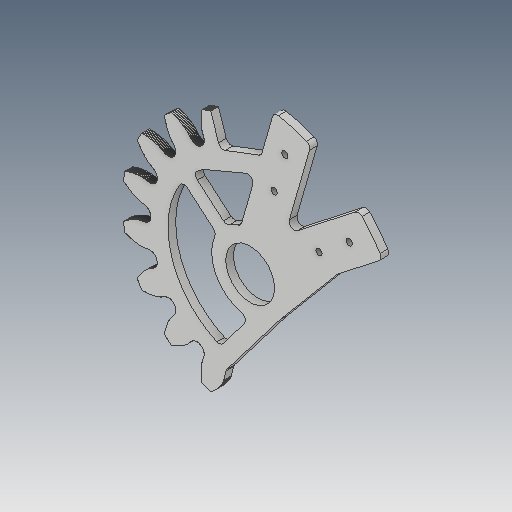
# Autodesk Inventor part: m5-18
Saved by Autodesk Inventor 2019.4 (Build 234330000, 330)
## iProperties
Created: 2019-06-11
Part Number: m5-18
Material: Generic
Document SubType Name: Modeling
Designer: AzLIer
Density: 1 g/cm^3
Appearance: Default
Mass: 10.3101 g
Surface Area: 90.7911 cm^2
Volume: 10.3101 cm^3
Autodesk Inventor part; units mm, degrees
(part 1 of 5)
ref_plane "YZ Plane" through (0, 0, 0) normal (1, 0, 0) x (0, 1, 0)
ref_plane "XZ Plane" through (0, 0, 0) normal (0, 1, 0) x (-1, 0, 0)
ref_plane "XY Plane" through (0, 0, 0) normal (0, 0, 1) x (1, 0, 0)
sketch "スケッチ1" plane through (0, 0, 0) normal (0, 0, 1) x (1, 0, 0)
  circle A0 centre (0, 0) radius 45 construction
  line L0 (-54, 0) -> (54, 0) construction
  line L1 (0, -54) -> (0, 54) construction
  line L2 (38.75, 0) -> (38.75, 0.0554)
  line L3 (38.75, 0.0554) -> (38.7498, 0.1108)
  line L4 (38.7498, 0.1108) -> (38.7496, 0.1663)
  line L5 (38.7496, 0.1663) -> (38.7494, 0.2217)
  line L6 (38.7494, 0.2217) -> (38.749, 0.2771)
  line L7 (38.749, 0.2771) -> (38.7743, 0.6234)
  line L8 (38.7743, 0.6234) -> (38.8288, 0.891)
  line L9 (38.8288, 0.891) -> (38.9042, 1.1194)
  line L10 (38.9042, 1.1194) -> (38.997, 1.3323)
  line L11 (38.997, 1.3323) -> (39.1059, 1.5242)
  line L12 (39.1059, 1.5242) -> (39.2291, 1.7067)
  line L13 (39.2291, 1.7067) -> (39.366, 1.8725)
  line L14 (39.366, 1.8725) -> (39.5158, 2.0289)
  line L15 (39.5158, 2.0289) -> (39.6781, 2.1727)
  line L16 (39.6781, 2.1727) -> (39.8523, 2.3033)
  line L17 (39.8523, 2.3033) -> (40.0379, 2.4272)
  line L18 (40.0379, 2.4272) -> (40.2348, 2.5371)
  line L19 (40.2348, 2.5371) -> (40.4428, 2.6351)
  line L20 (40.4428, 2.6351) -> (40.661, 2.7274)
  line L21 (40.661, 2.7274) -> (40.8898, 2.8078)
  line L22 (40.8898, 2.8078) -> (41.1289, 2.8764)
  line L23 (41.1289, 2.8764) -> (41.3781, 2.9334)
  line L24 (41.3781, 2.9334) -> (41.6367, 2.9845)
  line L25 (41.6367, 2.9845) -> (41.9049, 3.0266)
  line L26 (41.9049, 3.0266) -> (42.1825, 3.0578)
  line L27 (42.1825, 3.0578) -> (42.555, 3.1194)
  line L28 (42.555, 3.1194) -> (42.9254, 3.2087)
  line L29 (42.9254, 3.2087) -> (43.2942, 3.3167)
  line L30 (43.2942, 3.3167) -> (43.6617, 3.4402)
  line L31 (43.6617, 3.4402) -> (44.0279, 3.5774)
  line L32 (44.0279, 3.5774) -> (44.3927, 3.7271)
  line L33 (44.3927, 3.7271) -> (44.7563, 3.8884)
  line L34 (44.7563, 3.8884) -> (45.1184, 4.0607)
  line L35 (45.1184, 4.0607) -> (45.4792, 4.2434)
  line L36 (45.4792, 4.2434) -> (45.8385, 4.4362)
  line L37 (45.8385, 4.4362) -> (46.1963, 4.6386)
  line L38 (46.1963, 4.6386) -> (46.5526, 4.8504)
  line L39 (46.5526, 4.8504) -> (46.9072, 5.0713)
  line L40 (46.9072, 5.0713) -> (47.2601, 5.3011)
  line L41 (47.2601, 5.3011) -> (47.6113, 5.5395)
  line L42 (47.6113, 5.5395) -> (47.9606, 5.7865)
  line L43 (47.9606, 5.7865) -> (48.308, 6.0419)
  line L44 (48.308, 6.0419) -> (48.6534, 6.3055)
  line L45 (48.6534, 6.3055) -> (48.9968, 6.5771)
  line L46 (48.9968, 6.5771) -> (49.338, 6.8568)
  line L47 (49.338, 6.8568) -> (49.2867, 7.2162)
  line L48 (49.2867, 7.2162) -> (49.2328, 7.5752)
  line L49 (49.2328, 7.5752) -> (49.1763, 7.9338)
  line L50 (49.1763, 7.9338) -> (49.1172, 8.292)
  line L51 (49.1172, 8.292) -> (49.0554, 8.6498)
  circle A1 centre (0, 0) radius 45 construction
  line L52 (38.75, 0) -> (38.75, -0.0554)
  line L53 (38.75, -0.0554) -> (38.7498, -0.1108)
  line L54 (38.7498, -0.1108) -> (38.7496, -0.1663)
  line L55 (38.7496, -0.1663) -> (38.7494, -0.2217)
  line L56 (38.7494, -0.2217) -> (38.749, -0.2771)
  line L57 (38.749, -0.2771) -> (38.7743, -0.6234)
  line L58 (38.7743, -0.6234) -> (38.8288, -0.891)
  line L59 (38.8288, -0.891) -> (38.9042, -1.1194)
  line L60 (38.9042, -1.1194) -> (38.997, -1.3323)
  line L61 (38.997, -1.3323) -> (39.1059, -1.5242)
  line L62 (39.1059, -1.5242) -> (39.2291, -1.7067)
  line L63 (39.2291, -1.7067) -> (39.366, -1.8725)
  line L64 (39.366, -1.8725) -> (39.5158, -2.0289)
  line L65 (39.5158, -2.0289) -> (39.6781, -2.1727)
  line L66 (39.6781, -2.1727) -> (39.8523, -2.3033)
  line L67 (39.8523, -2.3033) -> (40.0379, -2.4272)
  line L68 (40.0379, -2.4272) -> (40.2348, -2.5371)
  line L69 (40.2348, -2.5371) -> (40.4428, -2.6351)
  line L70 (40.4428, -2.6351) -> (40.661, -2.7274)
  line L71 (40.661, -2.7274) -> (40.8898, -2.8078)
  line L72 (40.8898, -2.8078) -> (41.1289, -2.8764)
  line L73 (41.1289, -2.8764) -> (41.3781, -2.9334)
  line L74 (41.3781, -2.9334) -> (41.6367, -2.9845)
  line L75 (41.6367, -2.9845) -> (41.9049, -3.0266)
  line L76 (41.9049, -3.0266) -> (42.1825, -3.0578)
  line L77 (42.1825, -3.0578) -> (42.555, -3.1194)
  line L78 (42.555, -3.1194) -> (42.9254, -3.2087)
  line L79 (42.9254, -3.2087) -> (43.2942, -3.3167)
  line L80 (43.2942, -3.3167) -> (43.6617, -3.4402)
  line L81 (43.6617, -3.4402) -> (44.0279, -3.5774)
  line L82 (44.0279, -3.5774) -> (44.3927, -3.7271)
  line L83 (44.3927, -3.7271) -> (44.7563, -3.8884)
  line L84 (44.7563, -3.8884) -> (45.1184, -4.0607)
  line L85 (45.1184, -4.0607) -> (45.4792, -4.2434)
  line L86 (45.4792, -4.2434) -> (45.8385, -4.4362)
  line L87 (45.8385, -4.4362) -> (46.1963, -4.6386)
  line L88 (46.1963, -4.6386) -> (46.5526, -4.8504)
  line L89 (46.5526, -4.8504) -> (46.9072, -5.0713)
  line L90 (46.9072, -5.0713) -> (47.2601, -5.3011)
  line L91 (47.2601, -5.3011) -> (47.6113, -5.5395)
  line L92 (47.6113, -5.5395) -> (47.9606, -5.7865)
  line L93 (47.9606, -5.7865) -> (48.308, -6.0419)
  line L94 (48.308, -6.0419) -> (48.6534, -6.3055)
  line L95 (48.6534, -6.3055) -> (48.9968, -6.5771)
  line L96 (48.9968, -6.5771) -> (49.338, -6.8568)
  line L97 (49.338, -6.8568) -> (49.2867, -7.2162)
  line L98 (49.2867, -7.2162) -> (49.2328, -7.5752)
  line L99 (49.2328, -7.5752) -> (49.1763, -7.9338)
  line L100 (49.1763, -7.9338) -> (49.1172, -8.292)
  line L101 (49.1172, -8.292) -> (49.0554, -8.6498)
  line L102 (38.0283, 11.529) -> (38.2367, 11.4659)
  line L103 (38.2367, 11.4659) -> (38.4534, 11.4129)
  line L104 (38.4534, 11.4129) -> (38.6761, 11.377)
  line L105 (38.6761, 11.377) -> (38.905, 11.3561)
  line L106 (39.1417, 11.344) -> (39.3842, 11.3467)
  line L107 (39.3842, 11.3467) -> (39.6323, 11.364)
  line L108 (39.6323, 11.364) -> (39.886, 11.3956)
  line L109 (39.886, 11.3956) -> (40.1465, 11.4361)
  line L110 (40.1465, 11.4361) -> (40.4129, 11.4882)
  line L111 (36.4131, 13.2533) -> (36.3941, 13.3053)
  line L112 (36.3941, 13.3053) -> (36.375, 13.3574)
  line L113 (36.375, 13.3574) -> (36.3559, 13.4094)
  line L114 (36.3559, 13.4094) -> (36.3367, 13.4614)
  line L115 (40.6845, 11.5538) -> (41.0555, 11.6234)
  circle A2 centre (0, 0) radius 45 construction
  circle A3 centre (0, 0) radius 45 construction
  line L116 (36.3367, 13.4614) -> (36.3174, 13.5133)
  line L117 (36.3174, 13.5133) -> (36.2227, 13.8474)
  line L118 (36.2227, 13.8474) -> (36.1824, 14.1175)
  line L119 (36.1824, 14.1175) -> (36.1751, 14.3579)
  line L120 (36.1751, 14.3579) -> (36.1896, 14.5898)
  line L121 (36.1896, 14.5898) -> (36.2262, 14.8073)
  line L122 (36.2262, 14.8073) -> (36.2795, 15.0209)
  line L123 (36.2795, 15.0209) -> (36.3516, 15.2235)
  line L124 (36.3516, 15.2235) -> (36.4388, 15.4218)
  line L125 (36.4388, 15.4218) -> (36.5421, 15.6124)
  line L126 (36.5421, 15.6124) -> (36.6611, 15.7947)
  line L127 (36.6611, 15.7947) -> (36.7931, 15.9746)
  line L128 (36.7931, 15.9746) -> (36.9406, 16.1452)
  line L129 (36.9406, 16.1452) -> (37.1025, 16.3084)
  line L130 (37.1025, 16.3084) -> (37.2761, 16.4698)
  line L131 (40.4129, 11.4882) -> (40.6845, 11.5538)
  line L132 (37.2761, 16.4698) -> (37.4636, 16.6236)
  line L133 (37.4636, 16.6236) -> (37.6648, 16.7698)
  line L134 (37.6648, 16.7698) -> (37.8794, 16.9086)
  line L135 (37.8794, 16.9086) -> (38.105, 17.0451)
  line L136 (38.3425, 17.1764) -> (38.5928, 17.3007)
  line L137 (38.105, 17.0451) -> (38.3425, 17.1764)
  line L138 (38.905, 11.3561) -> (39.1417, 11.344)
  line L139 (38.5928, 17.3007) -> (38.9217, 17.4859)
  line L140 (38.9217, 17.4859) -> (39.2392, 17.6965)
  line L141 (39.5489, 17.9241) -> (39.852, 18.1659)
  line L142 (39.852, 18.1659) -> (40.1491, 18.4201)
  line L143 (40.1491, 18.4201) -> (40.4408, 18.6855)
  line L144 (39.2392, 17.6965) -> (39.5489, 17.9241)
  line L145 (37.8267, 11.6087) -> (38.0283, 11.529)
  line L146 (37.447, 11.8133) -> (37.6324, 11.7044)
  line L147 (37.6324, 11.7044) -> (37.8267, 11.6087)
  line L148 (40.7272, 18.9615) -> (41.0086, 19.2472)
  line L149 (42.5969, 21.1453) -> (42.8453, 21.4895)
  line L150 (42.3439, 20.8086) -> (42.5969, 21.1453)
  line L151 (42.0862, 20.4798) -> (42.3439, 20.8086)
  line L152 (41.8239, 20.1589) -> (42.0862, 20.4798)
  line L153 (41.5569, 19.8464) -> (41.8239, 20.1589)
  line L154 (41.2851, 19.5423) -> (41.5569, 19.8464)
  line L155 (41.0086, 19.2472) -> (41.2851, 19.5423)
  line L156 (42.8453, 21.4895) -> (43.0891, 21.841)
  line L157 (43.0891, 21.841) -> (43.3282, 22.1998)
  line L158 (43.3282, 22.1998) -> (43.5626, 22.5656)
  line L159 (43.5626, 22.5656) -> (43.7924, 22.9383)
  line L160 (43.7924, 22.9383) -> (44.0174, 23.3178)
  line L161 (44.0174, 23.3178) -> (43.8463, 23.638)
  line L162 (43.8463, 23.638) -> (43.6728, 23.957)
  line L163 (43.6728, 23.957) -> (43.4971, 24.2746)
  line L164 (43.4971, 24.2746) -> (43.319, 24.591)
  line L165 (43.319, 24.591) -> (43.1386, 24.9061)
  line L166 (40.4408, 18.6855) -> (40.7272, 18.9615)
  line L167 (37.2688, 11.9427) -> (37.447, 11.8133)
  line L168 (42.9903, 11.6809) -> (43.387, 11.6536)
  line L169 (42.5962, 11.6968) -> (42.9903, 11.6809)
  line L170 (42.2052, 11.7005) -> (42.5962, 11.6968)
  line L171 (41.8176, 11.6908) -> (42.2052, 11.7005)
  line L172 (41.4341, 11.6662) -> (41.8176, 11.6908)
  line L173 (41.0555, 11.6234) -> (41.4341, 11.6662)
  line L174 (43.387, 11.6536) -> (43.7863, 11.6156)
  line L175 (43.7863, 11.6156) -> (44.1878, 11.5673)
  line L176 (46.6346, 11.0786) -> (47.0473, 10.9659)
  line L177 (46.223, 11.1825) -> (46.6346, 11.0786)
  line L178 (45.8128, 11.2778) -> (46.223, 11.1825)
  line L179 (45.4041, 11.3641) -> (45.8128, 11.2778)
  line L180 (44.9969, 11.4412) -> (45.4041, 11.3641)
  line L181 (44.5914, 11.509) -> (44.9969, 11.4412)
  line L182 (44.1878, 11.5673) -> (44.5914, 11.509)
  line L183 (47.0473, 10.9659) -> (47.4611, 10.8448)
  line L184 (47.8758, 10.7152) -> (48.2914, 10.5774)
  line L185 (48.2914, 10.5774) -> (48.7077, 10.4313)
  line L186 (48.7077, 10.4313) -> (48.7824, 10.0761)
  line L187 (48.7824, 10.0761) -> (48.8546, 9.7203)
  line L188 (48.8546, 9.7203) -> (48.9241, 9.3639)
  line L189 (48.9241, 9.3639) -> (48.9911, 9.0071)
  line L190 (48.9911, 9.0071) -> (49.0554, 8.6498)
  line L191 (47.4611, 10.8448) -> (47.8758, 10.7152)
  line L192 (37.1009, 12.0858) -> (37.2688, 11.9427)
  line L193 (36.9408, 12.2541) -> (37.1009, 12.0858)
  line L194 (36.7919, 12.4429) -> (36.9408, 12.2541)
  line L195 (36.6492, 12.6758) -> (36.7919, 12.4429)
  line L196 (36.5069, 12.9926) -> (36.6492, 12.6758)
  line L197 (36.4883, 13.0448) -> (36.5069, 12.9926)
  line L198 (36.4696, 13.0969) -> (36.4883, 13.0448)
  line L199 (36.4508, 13.1491) -> (36.4696, 13.0969)
  line L200 (36.432, 13.2012) -> (36.4508, 13.1491)
  line L201 (36.4131, 13.2533) -> (36.432, 13.2012)
  line L202 (31.7918, 23.8401) -> (32.0092, 23.8521)
  line L203 (32.0092, 23.8521) -> (32.231, 23.8765)
  line L204 (32.231, 23.8765) -> (32.4525, 23.9189)
  line L205 (32.4525, 23.9189) -> (32.6748, 23.9775)
  line L206 (32.9013, 24.0471) -> (33.1282, 24.1326)
  line L207 (33.1282, 24.1326) -> (33.3555, 24.2337)
  line L208 (33.3555, 24.2337) -> (33.583, 24.3502)
  line L209 (33.583, 24.3502) -> (33.814, 24.4773)
  line L210 (33.814, 24.4773) -> (34.0465, 24.6174)
  line L211 (29.6842, 24.908) -> (29.6486, 24.9504)
  line L212 (29.6486, 24.9504) -> (29.6129, 24.9928)
  line L213 (29.6129, 24.9928) -> (29.5771, 25.0351)
  line L214 (29.5771, 25.0351) -> (29.5412, 25.0774)
  line L215 (34.2792, 24.772) -> (34.6041, 24.9642)
  circle A4 centre (0, 0) radius 45 construction
  circle A5 centre (0, 0) radius 45 construction
  line L216 (29.5412, 25.0774) -> (29.5054, 25.1196)
  line L217 (29.5054, 25.1196) -> (29.3021, 25.4012)
  line L218 (29.3021, 25.4012) -> (29.1718, 25.6412)
  line L219 (29.1718, 25.6412) -> (29.0828, 25.8646)
  line L220 (29.0828, 25.8646) -> (29.0171, 26.0875)
  line L221 (29.0171, 26.0875) -> (28.9771, 26.3044)
  line L222 (28.9771, 26.3044) -> (28.9541, 26.5234)
  line L223 (28.9541, 26.5234) -> (28.9525, 26.7384)
  line L224 (28.9525, 26.7384) -> (28.9667, 26.9545)
  line L225 (28.9667, 26.9545) -> (28.9985, 27.169)
  line L226 (28.9985, 27.169) -> (29.0481, 27.381)
  line L227 (29.0481, 27.381) -> (29.1106, 27.5952)
  line L228 (29.1106, 27.5952) -> (29.1908, 27.806)
  line L229 (29.1908, 27.806) -> (29.2872, 28.0147)
  line L230 (29.2872, 28.0147) -> (29.395, 28.2257)
  line L231 (34.0465, 24.6174) -> (34.2792, 24.772)
  line L232 (29.395, 28.2257) -> (29.5186, 28.4343)
  line L233 (29.5186, 28.4343) -> (29.6577, 28.6406)
  line L234 (29.6577, 28.6406) -> (29.8119, 28.8444)
  line L235 (29.8119, 28.8444) -> (29.9772, 29.0498)
  line L236 (30.1555, 29.2545) -> (30.3482, 29.4569)
  line L237 (29.9772, 29.0498) -> (30.1555, 29.2545)
  line L238 (32.6748, 23.9775) -> (32.9013, 24.0471)
  line L239 (30.3482, 29.4569) -> (30.5939, 29.7434)
  line L240 (30.5939, 29.7434) -> (30.8202, 30.0499)
  line L241 (31.0334, 30.3697) -> (31.2355, 30.7005)
  line L242 (31.2355, 30.7005) -> (31.4278, 31.041)
  line L243 (31.4278, 31.041) -> (31.6111, 31.3902)
  line L244 (30.8202, 30.0499) -> (31.0334, 30.3697)
  line L245 (31.575, 23.8461) -> (31.7918, 23.8401)
  line L246 (31.1483, 23.9085) -> (31.3597, 23.8696)
  line L247 (31.3597, 23.8696) -> (31.575, 23.8461)
  line L248 (31.7858, 31.7475) -> (31.9525, 32.1123)
  line L249 (32.7959, 34.4391) -> (32.9116, 34.8475)
  line L250 (32.6732, 34.0362) -> (32.7959, 34.4391)
  line L251 (32.5436, 33.639) -> (32.6732, 34.0362)
  line L252 (32.4068, 33.2478) -> (32.5436, 33.639)
  line L253 (32.2628, 32.8628) -> (32.4068, 33.2478)
  line L254 (32.1115, 32.4841) -> (32.2628, 32.8628)
  line L255 (31.9525, 32.1123) -> (32.1115, 32.4841)
  line L256 (32.9116, 34.8475) -> (33.0204, 35.2612)
  line L257 (33.0204, 35.2612) -> (33.1224, 35.6801)
  line L258 (33.1224, 35.6801) -> (33.2176, 36.1041)
  line L259 (33.2176, 36.1041) -> (33.306, 36.5329)
  line L260 (33.306, 36.5329) -> (33.3877, 36.9664)
  line L261 (33.3877, 36.9664) -> (33.1173, 37.2088)
  line L262 (33.1173, 37.2088) -> (32.8453, 37.4492)
  line L263 (32.8453, 37.4492) -> (32.5715, 37.6876)
  line L264 (32.5715, 37.6876) -> (32.2959, 37.924)
  line L265 (32.2959, 37.924) -> (32.0186, 38.1583)
  line L266 (31.6111, 31.3902) -> (31.7858, 31.7475)
  line L267 (30.9366, 23.9692) -> (31.1483, 23.9085)
  line L268 (36.4025, 25.68) -> (36.7847, 25.7901)
  line L269 (36.0268, 25.5601) -> (36.4025, 25.68)
  line L270 (35.6581, 25.4299) -> (36.0268, 25.5601)
  line L271 (35.2972, 25.2883) -> (35.6581, 25.4299)
  line L272 (34.9452, 25.1339) -> (35.2972, 25.2883)
  line L273 (34.6041, 24.9642) -> (34.9452, 25.1339)
  line L274 (36.7847, 25.7901) -> (37.1729, 25.8909)
  line L275 (37.1729, 25.8909) -> (37.5667, 25.9828)
  line L276 (40.0331, 26.3604) -> (40.4594, 26.3957)
  line L277 (39.6108, 26.3174) -> (40.0331, 26.3604)
  line L278 (39.1928, 26.2665) -> (39.6108, 26.3174)
  line L279 (38.7791, 26.2078) -> (39.1928, 26.2665)
  line L280 (38.3701, 26.1411) -> (38.7791, 26.2078)
  line L281 (37.9659, 26.0661) -> (38.3701, 26.1411)
  line L282 (37.5667, 25.9828) -> (37.9659, 26.0661)
  line L283 (40.4594, 26.3957) -> (40.8897, 26.4234)
  line L284 (41.3237, 26.4435) -> (41.7614, 26.4561)
  line L285 (41.7614, 26.4561) -> (42.2025, 26.4613)
  line L286 (42.2025, 26.4613) -> (42.3943, 26.153)
  line L287 (42.3943, 26.153) -> (42.5838, 25.8433)
  line L288 (42.5838, 25.8433) -> (42.771, 25.5322)
  line L289 (42.771, 25.5322) -> (42.9559, 25.2198)
  line L290 (42.9559, 25.2198) -> (43.1386, 24.9061)
  line L291 (40.8897, 26.4234) -> (41.3237, 26.4435)
  line L292 (30.7299, 24.0462) -> (30.9366, 23.9692)
  line L293 (30.5219, 24.1496) -> (30.7299, 24.0462)
  line L294 (30.3173, 24.2761) -> (30.5219, 24.1496)
  line L295 (30.1036, 24.4461) -> (30.3173, 24.2761)
  line L296 (29.8616, 24.6951) -> (30.1036, 24.4461)
  line L297 (29.8262, 24.7378) -> (29.8616, 24.6951)
  line L298 (29.7908, 24.7804) -> (29.8262, 24.7378)
  line L299 (29.7553, 24.823) -> (29.7908, 24.7804)
  line L300 (29.7198, 24.8655) -> (29.7553, 24.823)
  line L301 (29.6842, 24.908) -> (29.7198, 24.8655)
  line L302 (21.7207, 33.2758) -> (21.9209, 33.3615)
  line L303 (21.9209, 33.3615) -> (22.121, 33.4602)
  line L304 (22.121, 33.4602) -> (22.3146, 33.5758)
  line L305 (22.3146, 33.5758) -> (22.5034, 33.7069)
  line L306 (22.6925, 33.8498) -> (22.8765, 34.0078)
  line L307 (22.8765, 34.0078) -> (23.0555, 34.1805)
  line L308 (23.0555, 34.1805) -> (23.2294, 34.3678)
  line L309 (23.2294, 34.3678) -> (23.403, 34.5662)
  line L310 (23.403, 34.5662) -> (23.5736, 34.7774)
  line L311 (19.375, 33.5585) -> (19.327, 33.5862)
  line L312 (19.327, 33.5862) -> (19.2789, 33.6138)
  line L313 (19.2789, 33.6138) -> (19.2308, 33.6413)
  line L314 (19.2308, 33.6413) -> (19.1827, 33.6688)
  line L315 (23.7394, 35.0022) -> (23.979, 35.294)
  circle A6 centre (0, 0) radius 45 construction
  circle A7 centre (0, 0) radius 45 construction
  line L316 (19.1827, 33.6688) -> (19.1345, 33.6962)
  line L317 (19.1345, 33.6962) -> (18.8473, 33.8913)
  line L318 (18.8473, 33.8913) -> (18.6427, 34.0722)
  line L319 (18.6427, 34.0722) -> (18.4826, 34.2517)
  line L320 (18.4826, 34.2517) -> (18.3447, 34.4386)
  line L321 (18.3447, 34.4386) -> (18.2329, 34.6288)
  line L322 (18.2329, 34.6288) -> (18.1365, 34.8267)
  line L323 (18.1365, 34.8267) -> (18.0614, 35.0282)
  line L324 (18.0614, 35.0282) -> (18.0008, 35.2362)
  line L325 (18.0008, 35.2362) -> (17.9574, 35.4486)
  line L326 (17.9574, 35.4486) -> (17.9314, 35.6648)
  line L327 (17.9314, 35.6648) -> (17.9169, 35.8874)
  line L328 (17.9169, 35.8874) -> (17.9202, 36.1129)
  line L329 (17.9202, 36.1129) -> (17.9393, 36.342)
  line L330 (17.9393, 36.342) -> (17.9685, 36.5772)
  line L331 (23.5736, 34.7774) -> (23.7394, 35.0022)
  line L332 (17.9685, 36.5772) -> (18.0133, 36.8155)
  line L333 (18.0133, 36.8155) -> (18.0734, 37.0569)
  line L334 (18.0734, 37.0569) -> (18.1486, 37.3012)
  line L335 (18.1486, 37.3012) -> (18.2337, 37.5507)
  line L336 (18.3313, 37.804) -> (18.4431, 38.0601)
  line L337 (18.2337, 37.5507) -> (18.3313, 37.804)
  line L338 (22.5034, 33.7069) -> (22.6925, 33.8498)
  line L339 (18.4431, 38.0601) -> (18.576, 38.4134)
  line L340 (18.576, 38.4134) -> (18.6839, 38.7788)
  line L341 (18.7748, 39.1522) -> (18.8516, 39.5322)
  line L342 (18.8516, 39.5322) -> (18.9158, 39.9179)
  line L343 (18.9158, 39.9179) -> (18.9686, 40.3088)
  line L344 (18.6839, 38.7788) -> (18.7748, 39.1522)
  line L345 (21.515, 33.2073) -> (21.7207, 33.2758)
  line L346 (21.0926, 33.12) -> (21.3046, 33.1558)
  line L347 (21.3046, 33.1558) -> (21.515, 33.2073)
  line L348 (19.0107, 40.7043) -> (19.0425, 41.1041)
  line L349 (19.0392, 43.579) -> (19.0083, 44.0023)
  line L350 (19.0617, 43.1585) -> (19.0392, 43.579)
  line L351 (19.0757, 42.7409) -> (19.0617, 43.1585)
  line L352 (19.081, 42.3265) -> (19.0757, 42.7409)
  line L353 (19.0774, 41.9154) -> (19.081, 42.3265)
  line L354 (19.0647, 41.5079) -> (19.0774, 41.9154)
  line L355 (19.0425, 41.1041) -> (19.0647, 41.5079)
  line L356 (19.0083, 44.0023) -> (18.969, 44.4283)
  line L357 (18.969, 44.4283) -> (18.9216, 44.8569)
  line L358 (18.9216, 44.8569) -> (18.866, 45.2878)
  line L359 (18.866, 45.2878) -> (18.8024, 45.721)
  line L360 (18.8024, 45.721) -> (18.7309, 46.1563)
  line L361 (18.7309, 46.1563) -> (18.394, 46.2916)
  line L362 (18.394, 46.2916) -> (18.0561, 46.4245)
  line L363 (18.0561, 46.4245) -> (17.7172, 46.5548)
  line L364 (17.7172, 46.5548) -> (17.3775, 46.6827)
  line L365 (17.3775, 46.6827) -> (17.0368, 46.8081)
  line L366 (18.9686, 40.3088) -> (19.0107, 40.7043)
  line L367 (20.8729, 33.1046) -> (21.0926, 33.12)
  line L368 (25.4241, 36.5817) -> (25.7456, 36.8158)
  line L369 (25.1121, 36.3405) -> (25.4241, 36.5817)
  line L370 (24.8101, 36.092) -> (25.1121, 36.3405)
  line L371 (24.5194, 35.8356) -> (24.8101, 36.092)
  line L372 (24.2415, 35.5701) -> (24.5194, 35.8356)
  line L373 (23.979, 35.294) -> (24.2415, 35.5701)
  line L374 (25.7456, 36.8158) -> (26.0759, 37.0434)
  line L375 (26.0759, 37.0434) -> (26.4145, 37.2644)
  line L376 (28.603, 38.4628) -> (28.9916, 38.6418)
  line L377 (28.2209, 38.2779) -> (28.603, 38.4628)
  line L378 (27.8455, 38.0872) -> (28.2209, 38.2779)
  line L379 (27.4768, 37.8905) -> (27.8455, 38.0872)
  line L380 (27.1153, 37.6879) -> (27.4768, 37.8905)
  line L381 (26.7611, 37.4792) -> (27.1153, 37.6879)
  line L382 (26.4145, 37.2644) -> (26.7611, 37.4792)
  line L383 (28.9916, 38.6418) -> (29.3864, 38.815)
  line L384 (29.7874, 38.9823) -> (30.1943, 39.1439)
  line L385 (30.1943, 39.1439) -> (30.6071, 39.2996)
  line L386 (30.6071, 39.2996) -> (30.8927, 39.0755)
  line L387 (30.8927, 39.0755) -> (31.1767, 38.8493)
  line L388 (31.1767, 38.8493) -> (31.459, 38.621)
  line L389 (31.459, 38.621) -> (31.7397, 38.3907)
  line L390 (31.7397, 38.3907) -> (32.0186, 38.1583)
  line L391 (29.3864, 38.815) -> (29.7874, 38.9823)
  line L392 (20.6524, 33.1063) -> (20.8729, 33.1046)
  line L393 (20.4215, 33.1323) -> (20.6524, 33.1063)
  line L394 (20.186, 33.1812) -> (20.4215, 33.1323)
  line L395 (19.9271, 33.2679) -> (20.186, 33.1812)
  line L396 (19.6145, 33.4191) -> (19.9271, 33.2679)
  line L397 (19.5667, 33.4471) -> (19.6145, 33.4191)
  line L398 (19.5188, 33.475) -> (19.5667, 33.4471)
  line L399 (19.4709, 33.5029) -> (19.5188, 33.475)
  line L400 (19.423, 33.5307) -> (19.4709, 33.5029)
  line L401 (19.375, 33.5585) -> (19.423, 33.5307)
  line L402 (9.0298, 38.698) -> (9.1886, 38.8469)
  line L403 (9.1886, 38.8469) -> (9.3428, 39.0081)
  line L404 (9.3428, 39.0081) -> (9.4853, 39.183)
  line L405 (9.4853, 39.183) -> (9.6179, 39.3708)
  line L406 (9.7467, 39.5697) -> (9.8655, 39.7811)
  line L407 (9.8655, 39.7811) -> (9.9747, 40.0046)
  line L408 (9.9747, 40.0046) -> (10.0741, 40.2401)
  line L409 (10.0741, 40.2401) -> (10.1693, 40.4859)
  line L410 (10.1693, 40.4859) -> (10.2574, 40.7427)
  line L411 (6.7289, 38.1613) -> (6.6743, 38.1709)
  line L412 (6.6743, 38.1709) -> (6.6197, 38.1804)
  line L413 (6.6197, 38.1804) -> (6.5651, 38.1898)
  line L414 (6.5651, 38.1898) -> (6.5105, 38.1992)
  line L415 (10.3363, 41.0107) -> (10.4616, 41.3668)
  circle A8 centre (0, 0) radius 45 construction
  circle A9 centre (0, 0) radius 45 construction
  line L416 (6.5105, 38.1992) -> (6.4558, 38.2084)
  line L417 (6.4558, 38.2084) -> (6.1191, 38.2935)
  line L418 (6.1191, 38.2935) -> (5.8651, 38.3936)
  line L419 (5.8651, 38.3936) -> (5.6532, 38.5075)
  line L420 (5.6532, 38.5075) -> (5.4597, 38.636)
  line L421 (5.4597, 38.636) -> (5.2896, 38.7764)
  line L422 (5.2896, 38.7764) -> (5.1313, 38.9295)
  line L423 (5.1313, 38.9295) -> (4.9918, 39.0931)
  line L424 (4.9918, 39.0931) -> (4.8638, 39.2678)
  line L425 (4.8638, 39.2678) -> (4.7503, 39.4526)
  line L426 (4.7503, 39.4526) -> (4.6519, 39.6468)
  line L427 (4.6519, 39.6468) -> (4.5622, 39.8511)
  line L428 (4.5622, 39.8511) -> (4.4881, 40.0641)
  line L429 (4.4881, 40.0641) -> (4.4278, 40.2859)
  line L430 (4.4278, 40.2859) -> (4.3747, 40.5169)
  line L431 (10.2574, 40.7427) -> (10.3363, 41.0107)
  line L432 (4.3747, 40.5169) -> (4.3353, 40.7562)
  line L433 (4.3353, 40.7562) -> (4.3093, 41.0036)
  line L434 (4.3093, 41.0036) -> (4.2964, 41.2588)
  line L435 (4.2964, 41.2588) -> (4.291, 41.5224)
  line L436 (4.2961, 41.7938) -> (4.3135, 42.0727)
  line L437 (4.291, 41.5224) -> (4.2961, 41.7938)
  line L438 (9.6179, 39.3708) -> (9.7467, 39.5697)
  line L439 (4.3135, 42.0727) -> (4.3176, 42.4502)
  line L440 (4.3176, 42.4502) -> (4.294, 42.8304)
  line L441 (4.2517, 43.2124) -> (4.1939, 43.5958)
  line L442 (4.1939, 43.5958) -> (4.1223, 43.9802)
  line L443 (4.1223, 43.9802) -> (4.0382, 44.3655)
  line L444 (4.294, 42.8304) -> (4.2517, 43.2124)
  line L445 (8.8599, 38.5632) -> (9.0298, 38.698)
  line L446 (8.4928, 38.3367) -> (8.6799, 38.4428)
  line L447 (8.6799, 38.4428) -> (8.8599, 38.5632)
  line L448 (3.9425, 44.7515) -> (3.8357, 45.1381)
  line L449 (2.9861, 47.4626) -> (2.8122, 47.8499)
  line L450 (3.1511, 47.0752) -> (2.9861, 47.4626)
  line L451 (3.3071, 46.6876) -> (3.1511, 47.0752)
  line L452 (3.4538, 46.3) -> (3.3071, 46.6876)
  line L453 (3.591, 45.9125) -> (3.4538, 46.3)
  line L454 (3.7184, 45.5251) -> (3.591, 45.9125)
  line L455 (3.8357, 45.1381) -> (3.7184, 45.5251)
  line L456 (2.8122, 47.8499) -> (2.6297, 48.2368)
  line L457 (2.6297, 48.2368) -> (2.4385, 48.6232)
  line L458 (2.4385, 48.6232) -> (2.2389, 49.0092)
  line L459 (2.2389, 49.0092) -> (2.031, 49.3945)
  line L460 (2.031, 49.3945) -> (1.8149, 49.7791)
  line L461 (1.8149, 49.7791) -> (1.452, 49.791)
  line L462 (1.452, 49.791) -> (1.0891, 49.8003)
  line L463 (1.0891, 49.8003) -> (0.7261, 49.8069)
  line L464 (0.7261, 49.8069) -> (0.363, 49.8108)
  line L465 (0.363, 49.8108) -> (0, 49.8122)
  line L466 (4.0382, 44.3655) -> (3.9425, 44.7515)
  line L467 (8.2917, 38.2471) -> (8.4928, 38.3367)
  line L468 (11.3792, 43.0711) -> (11.6012, 43.4011)
  line L469 (11.1684, 42.7378) -> (11.3792, 43.0711)
  line L470 (10.9697, 42.401) -> (11.1684, 42.7378)
  line L471 (10.7842, 42.0605) -> (10.9697, 42.401)
  line L472 (10.6138, 41.716) -> (10.7842, 42.0605)
  line L473 (10.4616, 41.3668) -> (10.6138, 41.716)
  line L474 (11.6012, 43.4011) -> (11.8338, 43.7278)
  line L475 (11.8338, 43.7278) -> (12.0764, 44.0514)
  line L476 (13.723, 45.926) -> (14.0269, 46.2271)
  line L477 (13.4272, 45.6216) -> (13.723, 45.926)
  line L478 (13.1396, 45.314) -> (13.4272, 45.6216)
  line L479 (12.8605, 45.0031) -> (13.1396, 45.314)
  line L480 (12.59, 44.689) -> (12.8605, 45.0031)
  line L481 (12.3286, 44.3718) -> (12.59, 44.689)
  line L482 (12.0764, 44.0514) -> (12.3286, 44.3718)
  line L483 (14.0269, 46.2271) -> (14.3387, 46.5249)
  line L484 (14.6582, 46.8193) -> (14.9854, 47.1103)
  line L485 (14.9854, 47.1103) -> (15.32, 47.3978)
  line L486 (15.32, 47.3978) -> (15.6651, 47.2849)
  line L487 (15.6651, 47.2849) -> (16.0093, 47.1694)
  line L488 (16.0093, 47.1694) -> (16.3527, 47.0515)
  line L489 (16.3527, 47.0515) -> (16.6952, 46.9311)
  line L490 (16.6952, 46.9311) -> (17.0368, 46.8081)
  line L491 (14.3387, 46.5249) -> (14.6582, 46.8193)
  line L492 (8.0839, 38.1732) -> (8.2917, 38.2471)
  line L493 (7.8581, 38.1187) -> (8.0839, 38.1732)
  line L494 (7.62, 38.0842) -> (7.8581, 38.1187)
  line L495 (7.347, 38.077) -> (7.62, 38.0842)
  line L496 (7.0016, 38.1122) -> (7.347, 38.077)
  line L497 (6.9471, 38.1222) -> (7.0016, 38.1122)
  line L498 (6.8925, 38.1321) -> (6.9471, 38.1222)
  line L499 (6.838, 38.1419) -> (6.8925, 38.1321)
  line L500 (6.7834, 38.1516) -> (6.838, 38.1419)
  line L501 (6.7289, 38.1613) -> (6.7834, 38.1516)
  line L502 (-4.7503, 39.4526) -> (-4.6519, 39.6468)
  line L503 (-4.6519, 39.6468) -> (-4.5622, 39.8511)
  line L504 (-4.5622, 39.8511) -> (-4.4881, 40.0641)
  line L505 (-4.4881, 40.0641) -> (-4.4278, 40.2859)
  line L506 (-4.3747, 40.5169) -> (-4.3353, 40.7562)
  line L507 (-4.3353, 40.7562) -> (-4.3093, 41.0036)
  line L508 (-4.3093, 41.0036) -> (-4.2964, 41.2588)
  line L509 (-4.2964, 41.2588) -> (-4.291, 41.5224)
  line L510 (-4.291, 41.5224) -> (-4.2961, 41.7938)
  line L511 (-6.7289, 38.1613) -> (-6.7834, 38.1516)
  line L512 (-6.7834, 38.1516) -> (-6.838, 38.1419)
  line L513 (-6.838, 38.1419) -> (-6.8925, 38.1321)
  line L514 (-6.8925, 38.1321) -> (-6.9471, 38.1222)
  line L515 (-4.3135, 42.0727) -> (-4.3176, 42.4502)
  circle A10 centre (0, 0) radius 45 construction
  circle A11 centre (0, 0) radius 45 construction
  line L516 (-6.9471, 38.1222) -> (-7.0016, 38.1122)
  line L517 (-7.0016, 38.1122) -> (-7.347, 38.077)
  line L518 (-7.347, 38.077) -> (-7.62, 38.0842)
  line L519 (-7.62, 38.0842) -> (-7.8581, 38.1187)
  line L520 (-7.8581, 38.1187) -> (-8.0839, 38.1732)
  line L521 (-8.0839, 38.1732) -> (-8.2917, 38.2471)
  line L522 (-8.2917, 38.2471) -> (-8.4928, 38.3367)
  line L523 (-8.4928, 38.3367) -> (-8.6799, 38.4428)
  line L524 (-8.6799, 38.4428) -> (-8.8599, 38.5632)
  line L525 (-8.8599, 38.5632) -> (-9.0298, 38.698)
  line L526 (-9.0298, 38.698) -> (-9.1886, 38.8469)
  line L527 (-9.1886, 38.8469) -> (-9.3428, 39.0081)
  line L528 (-9.3428, 39.0081) -> (-9.4853, 39.183)
  line L529 (-9.4853, 39.183) -> (-9.6179, 39.3708)
  line L530 (-9.6179, 39.3708) -> (-9.7467, 39.5697)
  line L531 (-4.2961, 41.7938) -> (-4.3135, 42.0727)
  line L532 (-9.7467, 39.5697) -> (-9.8655, 39.7811)
  line L533 (-9.8655, 39.7811) -> (-9.9747, 40.0046)
  line L534 (-9.9747, 40.0046) -> (-10.0741, 40.2401)
  line L535 (-10.0741, 40.2401) -> (-10.1693, 40.4859)
  line L536 (-10.2574, 40.7427) -> (-10.3363, 41.0107)
  line L537 (-10.1693, 40.4859) -> (-10.2574, 40.7427)
  line L538 (-4.4278, 40.2859) -> (-4.3747, 40.5169)
  line L539 (-10.3363, 41.0107) -> (-10.4616, 41.3668)
  line L540 (-10.4616, 41.3668) -> (-10.6138, 41.716)
  line L541 (-10.7842, 42.0605) -> (-10.9697, 42.401)
  line L542 (-10.9697, 42.401) -> (-11.1684, 42.7378)
  line L543 (-11.1684, 42.7378) -> (-11.3792, 43.0711)
  line L544 (-10.6138, 41.716) -> (-10.7842, 42.0605)
  line L545 (-4.8638, 39.2678) -> (-4.7503, 39.4526)
  line L546 (-5.1313, 38.9295) -> (-4.9918, 39.0931)
  line L547 (-4.9918, 39.0931) -> (-4.8638, 39.2678)
  line L548 (-11.6012, 43.4011) -> (-11.8338, 43.7278)
  line L549 (-13.4272, 45.6216) -> (-13.723, 45.926)
  line L550 (-13.1396, 45.314) -> (-13.4272, 45.6216)
  line L551 (-12.8605, 45.0031) -> (-13.1396, 45.314)
  line L552 (-12.59, 44.689) -> (-12.8605, 45.0031)
  line L553 (-12.3286, 44.3718) -> (-12.59, 44.689)
  line L554 (-12.0764, 44.0514) -> (-12.3286, 44.3718)
  line L555 (-11.8338, 43.7278) -> (-12.0764, 44.0514)
  line L556 (-13.723, 45.926) -> (-14.0269, 46.2271)
  line L557 (-14.0269, 46.2271) -> (-14.3387, 46.5249)
  line L558 (-14.3387, 46.5249) -> (-14.6582, 46.8193)
  line L559 (-14.6582, 46.8193) -> (-14.9854, 47.1103)
  line L560 (-14.9854, 47.1103) -> (-15.32, 47.3978)
  line L561 (-15.32, 47.3978) -> (-15.6651, 47.2849)
  line L562 (-15.6651, 47.2849) -> (-16.0093, 47.1694)
  line L563 (-16.0093, 47.1694) -> (-16.3527, 47.0515)
  line L564 (-16.3527, 47.0515) -> (-16.6952, 46.9311)
  line L565 (-16.6952, 46.9311) -> (-17.0368, 46.8081)
  line L566 (-11.3792, 43.0711) -> (-11.6012, 43.4011)
  line L567 (-5.2896, 38.7764) -> (-5.1313, 38.9295)
  line L568 (-4.0382, 44.3655) -> (-3.9425, 44.7515)
  line L569 (-4.1223, 43.9802) -> (-4.0382, 44.3655)
  line L570 (-4.1939, 43.5958) -> (-4.1223, 43.9802)
  line L571 (-4.2517, 43.2124) -> (-4.1939, 43.5958)
  line L572 (-4.294, 42.8304) -> (-4.2517, 43.2124)
  line L573 (-4.3176, 42.4502) -> (-4.294, 42.8304)
  line L574 (-3.9425, 44.7515) -> (-3.8357, 45.1381)
  line L575 (-3.8357, 45.1381) -> (-3.7184, 45.5251)
  line L576 (-2.8122, 47.8499) -> (-2.6297, 48.2368)
  line L577 (-2.9861, 47.4626) -> (-2.8122, 47.8499)
  line L578 (-3.1511, 47.0752) -> (-2.9861, 47.4626)
  line L579 (-3.3071, 46.6876) -> (-3.1511, 47.0752)
  line L580 (-3.4538, 46.3) -> (-3.3071, 46.6876)
  line L581 (-3.591, 45.9125) -> (-3.4538, 46.3)
  line L582 (-3.7184, 45.5251) -> (-3.591, 45.9125)
  line L583 (-2.6297, 48.2368) -> (-2.4385, 48.6232)
  line L584 (-2.2389, 49.0092) -> (-2.031, 49.3945)
  line L585 (-2.031, 49.3945) -> (-1.8149, 49.7791)
  line L586 (-1.8149, 49.7791) -> (-1.452, 49.791)
  line L587 (-1.452, 49.791) -> (-1.0891, 49.8003)
  line L588 (-1.0891, 49.8003) -> (-0.7261, 49.8069)
  line L589 (-0.7261, 49.8069) -> (-0.363, 49.8108)
  line L590 (-0.363, 49.8108) -> (0, 49.8122)
  line L591 (-2.4385, 48.6232) -> (-2.2389, 49.0092)
  line L592 (-5.4597, 38.636) -> (-5.2896, 38.7764)
  line L593 (-5.6532, 38.5075) -> (-5.4597, 38.636)
  line L594 (-5.8651, 38.3936) -> (-5.6532, 38.5075)
  line L595 (-6.1191, 38.2935) -> (-5.8651, 38.3936)
  line L596 (-6.4558, 38.2084) -> (-6.1191, 38.2935)
  line L597 (-6.5105, 38.1992) -> (-6.4558, 38.2084)
  line L598 (-6.5651, 38.1898) -> (-6.5105, 38.1992)
  line L599 (-6.6197, 38.1804) -> (-6.5651, 38.1898)
  line L600 (-6.6743, 38.1709) -> (-6.6197, 38.1804)
  line L601 (-6.7289, 38.1613) -> (-6.6743, 38.1709)
  line L602 (-17.9574, 35.4486) -> (-17.9314, 35.6648)
  line L603 (-17.9314, 35.6648) -> (-17.9169, 35.8874)
  line L604 (-17.9169, 35.8874) -> (-17.9202, 36.1129)
  line L605 (-17.9202, 36.1129) -> (-17.9393, 36.342)
  line L606 (-17.9685, 36.5772) -> (-18.0133, 36.8155)
  line L607 (-18.0133, 36.8155) -> (-18.0734, 37.0569)
  line L608 (-18.0734, 37.0569) -> (-18.1486, 37.3012)
  line L609 (-18.1486, 37.3012) -> (-18.2337, 37.5507)
  line L610 (-18.2337, 37.5507) -> (-18.3313, 37.804)
  line L611 (-19.375, 33.5585) -> (-19.423, 33.5307)
  line L612 (-19.423, 33.5307) -> (-19.4709, 33.5029)
  line L613 (-19.4709, 33.5029) -> (-19.5188, 33.475)
  line L614 (-19.5188, 33.475) -> (-19.5667, 33.4471)
  line L615 (-18.4431, 38.0601) -> (-18.576, 38.4134)
  circle A12 centre (0, 0) radius 45 construction
  circle A13 centre (0, 0) radius 45 construction
  line L616 (-19.5667, 33.4471) -> (-19.6145, 33.4191)
  line L617 (-19.6145, 33.4191) -> (-19.9271, 33.2679)
  line L618 (-19.9271, 33.2679) -> (-20.186, 33.1812)
  line L619 (-20.186, 33.1812) -> (-20.4215, 33.1323)
  line L620 (-20.4215, 33.1323) -> (-20.6524, 33.1063)
  line L621 (-20.6524, 33.1063) -> (-20.8729, 33.1046)
  line L622 (-20.8729, 33.1046) -> (-21.0926, 33.12)
  line L623 (-21.0926, 33.12) -> (-21.3046, 33.1558)
  line L624 (-21.3046, 33.1558) -> (-21.515, 33.2073)
  line L625 (-21.515, 33.2073) -> (-21.7207, 33.2758)
  line L626 (-21.7207, 33.2758) -> (-21.9209, 33.3615)
  line L627 (-21.9209, 33.3615) -> (-22.121, 33.4602)
  line L628 (-22.121, 33.4602) -> (-22.3146, 33.5758)
  line L629 (-22.3146, 33.5758) -> (-22.5034, 33.7069)
  line L630 (-22.5034, 33.7069) -> (-22.6925, 33.8498)
  line L631 (-18.3313, 37.804) -> (-18.4431, 38.0601)
  line L632 (-22.6925, 33.8498) -> (-22.8765, 34.0078)
  line L633 (-22.8765, 34.0078) -> (-23.0555, 34.1805)
  line L634 (-23.0555, 34.1805) -> (-23.2294, 34.3678)
  line L635 (-23.2294, 34.3678) -> (-23.403, 34.5662)
  line L636 (-23.5736, 34.7774) -> (-23.7394, 35.0022)
  line L637 (-23.403, 34.5662) -> (-23.5736, 34.7774)
  line L638 (-17.9393, 36.342) -> (-17.9685, 36.5772)
  line L639 (-23.7394, 35.0022) -> (-23.979, 35.294)
  line L640 (-23.979, 35.294) -> (-24.2415, 35.5701)
  line L641 (-24.5194, 35.8356) -> (-24.8101, 36.092)
  line L642 (-24.8101, 36.092) -> (-25.1121, 36.3405)
  line L643 (-25.1121, 36.3405) -> (-25.4241, 36.5817)
  line L644 (-24.2415, 35.5701) -> (-24.5194, 35.8356)
  line L645 (-18.0008, 35.2362) -> (-17.9574, 35.4486)
  line L646 (-18.1365, 34.8267) -> (-18.0614, 35.0282)
  line L647 (-18.0614, 35.0282) -> (-18.0008, 35.2362)
  line L648 (-25.7456, 36.8158) -> (-26.0759, 37.0434)
  line L649 (-28.2209, 38.2779) -> (-28.603, 38.4628)
  line L650 (-27.8455, 38.0872) -> (-28.2209, 38.2779)
  line L651 (-27.4768, 37.8905) -> (-27.8455, 38.0872)
  line L652 (-27.1153, 37.6879) -> (-27.4768, 37.8905)
  line L653 (-26.7611, 37.4792) -> (-27.1153, 37.6879)
  line L654 (-26.4145, 37.2644) -> (-26.7611, 37.4792)
  line L655 (-26.0759, 37.0434) -> (-26.4145, 37.2644)
  line L656 (-28.603, 38.4628) -> (-28.9916, 38.6418)
  line L657 (-28.9916, 38.6418) -> (-29.3864, 38.815)
  line L658 (-29.3864, 38.815) -> (-29.7874, 38.9823)
  line L659 (-29.7874, 38.9823) -> (-30.1943, 39.1439)
  line L660 (-30.1943, 39.1439) -> (-30.6071, 39.2996)
  line L661 (-30.6071, 39.2996) -> (-30.8927, 39.0755)
  line L662 (-30.8927, 39.0755) -> (-31.1767, 38.8493)
  line L663 (-31.1767, 38.8493) -> (-31.459, 38.621)
  line L664 (-31.459, 38.621) -> (-31.7397, 38.3907)
  line L665 (-31.7397, 38.3907) -> (-32.0186, 38.1583)
  line L666 (-25.4241, 36.5817) -> (-25.7456, 36.8158)
  line L667 (-18.2329, 34.6288) -> (-18.1365, 34.8267)
  line L668 (-18.9686, 40.3088) -> (-19.0107, 40.7043)
  line L669 (-18.9158, 39.9179) -> (-18.9686, 40.3088)
  line L670 (-18.8516, 39.5322) -> (-18.9158, 39.9179)
  line L671 (-18.7748, 39.1522) -> (-18.8516, 39.5322)
  line L672 (-18.6839, 38.7788) -> (-18.7748, 39.1522)
  line L673 (-18.576, 38.4134) -> (-18.6839, 38.7788)
  line L674 (-19.0107, 40.7043) -> (-19.0425, 41.1041)
  line L675 (-19.0425, 41.1041) -> (-19.0647, 41.5079)
  line L676 (-19.0083, 44.0023) -> (-18.969, 44.4283)
  line L677 (-19.0392, 43.579) -> (-19.0083, 44.0023)
  line L678 (-19.0617, 43.1585) -> (-19.0392, 43.579)
  line L679 (-19.0757, 42.7409) -> (-19.0617, 43.1585)
  line L680 (-19.081, 42.3265) -> (-19.0757, 42.7409)
  line L681 (-19.0774, 41.9154) -> (-19.081, 42.3265)
  line L682 (-19.0647, 41.5079) -> (-19.0774, 41.9154)
  line L683 (-18.969, 44.4283) -> (-18.9216, 44.8569)
  line L684 (-18.866, 45.2878) -> (-18.8024, 45.721)
  line L685 (-18.8024, 45.721) -> (-18.7309, 46.1563)
  line L686 (-18.7309, 46.1563) -> (-18.394, 46.2916)
  line L687 (-18.394, 46.2916) -> (-18.0561, 46.4245)
  line L688 (-18.0561, 46.4245) -> (-17.7172, 46.5548)
  line L689 (-17.7172, 46.5548) -> (-17.3775, 46.6827)
  line L690 (-17.3775, 46.6827) -> (-17.0368, 46.8081)
  line L691 (-18.9216, 44.8569) -> (-18.866, 45.2878)
  line L692 (-18.3447, 34.4386) -> (-18.2329, 34.6288)
  line L693 (-18.4826, 34.2517) -> (-18.3447, 34.4386)
  line L694 (-18.6427, 34.0722) -> (-18.4826, 34.2517)
  line L695 (-18.8473, 33.8913) -> (-18.6427, 34.0722)
  line L696 (-19.1345, 33.6962) -> (-18.8473, 33.8913)
  line L697 (-19.1827, 33.6688) -> (-19.1345, 33.6962)
  line L698 (-19.2308, 33.6413) -> (-19.1827, 33.6688)
  line L699 (-19.2789, 33.6138) -> (-19.2308, 33.6413)
  line L700 (-19.327, 33.5862) -> (-19.2789, 33.6138)
  line L701 (-19.375, 33.5585) -> (-19.327, 33.5862)
  line L702 (-28.9985, 27.169) -> (-29.0481, 27.381)
  line L703 (-29.0481, 27.381) -> (-29.1106, 27.5952)
  line L704 (-29.1106, 27.5952) -> (-29.1908, 27.806)
  line L705 (-29.1908, 27.806) -> (-29.2872, 28.0147)
  line L706 (-29.395, 28.2257) -> (-29.5186, 28.4343)
  line L707 (-29.5186, 28.4343) -> (-29.6577, 28.6406)
  line L708 (-29.6577, 28.6406) -> (-29.8119, 28.8444)
  line L709 (-29.8119, 28.8444) -> (-29.9772, 29.0498)
  line L710 (-29.9772, 29.0498) -> (-30.1555, 29.2545)
  line L711 (-29.6842, 24.908) -> (-29.7198, 24.8655)
  line L712 (-29.7198, 24.8655) -> (-29.7553, 24.823)
  line L713 (-29.7553, 24.823) -> (-29.7908, 24.7804)
  line L714 (-29.7908, 24.7804) -> (-29.8262, 24.7378)
  line L715 (-30.3482, 29.4569) -> (-30.5939, 29.7434)
  circle A14 centre (0, 0) radius 45 construction
  circle A15 centre (0, 0) radius 45 construction
  line L716 (-29.8262, 24.7378) -> (-29.8616, 24.6951)
  line L717 (-29.8616, 24.6951) -> (-30.1036, 24.4461)
  line L718 (-30.1036, 24.4461) -> (-30.3173, 24.2761)
  line L719 (-30.3173, 24.2761) -> (-30.5219, 24.1496)
  line L720 (-30.5219, 24.1496) -> (-30.7299, 24.0462)
  line L721 (-30.7299, 24.0462) -> (-30.9366, 23.9692)
  line L722 (-30.9366, 23.9692) -> (-31.1483, 23.9085)
  line L723 (-31.1483, 23.9085) -> (-31.3597, 23.8696)
  line L724 (-31.3597, 23.8696) -> (-31.575, 23.8461)
  line L725 (-31.575, 23.8461) -> (-31.7918, 23.8401)
  line L726 (-31.7918, 23.8401) -> (-32.0092, 23.8521)
  line L727 (-32.0092, 23.8521) -> (-32.231, 23.8765)
  line L728 (-32.231, 23.8765) -> (-32.4525, 23.9189)
  line L729 (-32.4525, 23.9189) -> (-32.6748, 23.9775)
  line L730 (-32.6748, 23.9775) -> (-32.9013, 24.0471)
  line L731 (-30.1555, 29.2545) -> (-30.3482, 29.4569)
  line L732 (-32.9013, 24.0471) -> (-33.1282, 24.1326)
  line L733 (-33.1282, 24.1326) -> (-33.3555, 24.2337)
  line L734 (-33.3555, 24.2337) -> (-33.583, 24.3502)
  line L735 (-33.583, 24.3502) -> (-33.814, 24.4773)
  line L736 (-34.0465, 24.6174) -> (-34.2792, 24.772)
  line L737 (-33.814, 24.4773) -> (-34.0465, 24.6174)
  line L738 (-29.2872, 28.0147) -> (-29.395, 28.2257)
  line L739 (-34.2792, 24.772) -> (-34.6041, 24.9642)
  line L740 (-34.6041, 24.9642) -> (-34.9452, 25.1339)
  line L741 (-35.2972, 25.2883) -> (-35.6581, 25.4299)
  line L742 (-35.6581, 25.4299) -> (-36.0268, 25.5601)
  line L743 (-36.0268, 25.5601) -> (-36.4025, 25.68)
  line L744 (-34.9452, 25.1339) -> (-35.2972, 25.2883)
  line L745 (-28.9667, 26.9545) -> (-28.9985, 27.169)
  line L746 (-28.9541, 26.5234) -> (-28.9525, 26.7384)
  line L747 (-28.9525, 26.7384) -> (-28.9667, 26.9545)
  line L748 (-36.7847, 25.7901) -> (-37.1729, 25.8909)
  line L749 (-39.6108, 26.3174) -> (-40.0331, 26.3604)
  line L750 (-39.1928, 26.2665) -> (-39.6108, 26.3174)
  line L751 (-38.7791, 26.2078) -> (-39.1928, 26.2665)
  line L752 (-38.3701, 26.1411) -> (-38.7791, 26.2078)
  line L753 (-37.9659, 26.0661) -> (-38.3701, 26.1411)
  line L754 (-37.5667, 25.9828) -> (-37.9659, 26.0661)
  line L755 (-37.1729, 25.8909) -> (-37.5667, 25.9828)
  line L756 (-40.0331, 26.3604) -> (-40.4594, 26.3957)
  line L757 (-40.4594, 26.3957) -> (-40.8897, 26.4234)
  line L758 (-40.8897, 26.4234) -> (-41.3237, 26.4435)
  line L759 (-41.3237, 26.4435) -> (-41.7614, 26.4561)
  line L760 (-41.7614, 26.4561) -> (-42.2025, 26.4613)
  line L761 (-42.2025, 26.4613) -> (-42.3943, 26.153)
  line L762 (-42.3943, 26.153) -> (-42.5838, 25.8433)
  line L763 (-42.5838, 25.8433) -> (-42.771, 25.5322)
  line L764 (-42.771, 25.5322) -> (-42.9559, 25.2198)
  line L765 (-42.9559, 25.2198) -> (-43.1386, 24.9061)
  line L766 (-36.4025, 25.68) -> (-36.7847, 25.7901)
  line L767 (-28.9771, 26.3044) -> (-28.9541, 26.5234)
  line L768 (-31.6111, 31.3902) -> (-31.7858, 31.7475)
  line L769 (-31.4278, 31.041) -> (-31.6111, 31.3902)
  line L770 (-31.2355, 30.7005) -> (-31.4278, 31.041)
  line L771 (-31.0334, 30.3697) -> (-31.2355, 30.7005)
  line L772 (-30.8202, 30.0499) -> (-31.0334, 30.3697)
  line L773 (-30.5939, 29.7434) -> (-30.8202, 30.0499)
  line L774 (-31.7858, 31.7475) -> (-31.9525, 32.1123)
  line L775 (-31.9525, 32.1123) -> (-32.1115, 32.4841)
  line L776 (-32.9116, 34.8475) -> (-33.0204, 35.2612)
  line L777 (-32.7959, 34.4391) -> (-32.9116, 34.8475)
  line L778 (-32.6732, 34.0362) -> (-32.7959, 34.4391)
  line L779 (-32.5436, 33.639) -> (-32.6732, 34.0362)
  line L780 (-32.4068, 33.2478) -> (-32.5436, 33.639)
  line L781 (-32.2628, 32.8628) -> (-32.4068, 33.2478)
  line L782 (-32.1115, 32.4841) -> (-32.2628, 32.8628)
  line L783 (-33.0204, 35.2612) -> (-33.1224, 35.6801)
  line L784 (-33.2176, 36.1041) -> (-33.306, 36.5329)
  line L785 (-33.306, 36.5329) -> (-33.3877, 36.9664)
  line L786 (-33.3877, 36.9664) -> (-33.1173, 37.2088)
  line L787 (-33.1173, 37.2088) -> (-32.8453, 37.4492)
  line L788 (-32.8453, 37.4492) -> (-32.5715, 37.6876)
  line L789 (-32.5715, 37.6876) -> (-32.2959, 37.924)
  line L790 (-32.2959, 37.924) -> (-32.0186, 38.1583)
  line L791 (-33.1224, 35.6801) -> (-33.2176, 36.1041)
  line L792 (-29.0171, 26.0875) -> (-28.9771, 26.3044)
  line L793 (-29.0828, 25.8646) -> (-29.0171, 26.0875)
  line L794 (-29.1718, 25.6412) -> (-29.0828, 25.8646)
  line L795 (-29.3021, 25.4012) -> (-29.1718, 25.6412)
  line L796 (-29.5054, 25.1196) -> (-29.3021, 25.4012)
  line L797 (-29.5412, 25.0774) -> (-29.5054, 25.1196)
  line L798 (-29.5771, 25.0351) -> (-29.5412, 25.0774)
  line L799 (-29.6129, 24.9928) -> (-29.5771, 25.0351)
  line L800 (-29.6486, 24.9504) -> (-29.6129, 24.9928)
  line L801 (-29.6842, 24.908) -> (-29.6486, 24.9504)
  line L802 (-36.5421, 15.6124) -> (-36.6611, 15.7947)
  line L803 (-36.6611, 15.7947) -> (-36.7931, 15.9746)
  line L804 (-36.7931, 15.9746) -> (-36.9406, 16.1452)
  line L805 (-36.9406, 16.1452) -> (-37.1025, 16.3084)
  line L806 (-37.2761, 16.4698) -> (-37.4636, 16.6236)
  line L807 (-37.4636, 16.6236) -> (-37.6648, 16.7698)
  line L808 (-37.6648, 16.7698) -> (-37.8794, 16.9086)
  line L809 (-37.8794, 16.9086) -> (-38.105, 17.0451)
  line L810 (-38.105, 17.0451) -> (-38.3425, 17.1764)
  line L811 (-36.4131, 13.2533) -> (-36.432, 13.2012)
  line L812 (-36.432, 13.2012) -> (-36.4508, 13.1491)
  line L813 (-36.4508, 13.1491) -> (-36.4696, 13.0969)
  line L814 (-36.4696, 13.0969) -> (-36.4883, 13.0448)
  line L815 (-38.5928, 17.3007) -> (-38.9217, 17.4859)
  circle A16 centre (0, 0) radius 45 construction
  circle A17 centre (0, 0) radius 45 construction
  line L816 (-36.4883, 13.0448) -> (-36.5069, 12.9926)
  line L817 (-36.5069, 12.9926) -> (-36.6492, 12.6758)
  line L818 (-36.6492, 12.6758) -> (-36.7919, 12.4429)
  line L819 (-36.7919, 12.4429) -> (-36.9408, 12.2541)
  line L820 (-36.9408, 12.2541) -> (-37.1009, 12.0858)
  line L821 (-37.1009, 12.0858) -> (-37.2688, 11.9427)
  line L822 (-37.2688, 11.9427) -> (-37.447, 11.8133)
  line L823 (-37.447, 11.8133) -> (-37.6324, 11.7044)
  line L824 (-37.6324, 11.7044) -> (-37.8267, 11.6087)
  line L825 (-37.8267, 11.6087) -> (-38.0283, 11.529)
  line L826 (-38.0283, 11.529) -> (-38.2367, 11.4659)
  line L827 (-38.2367, 11.4659) -> (-38.4534, 11.4129)
  line L828 (-38.4534, 11.4129) -> (-38.6761, 11.377)
  line L829 (-38.6761, 11.377) -> (-38.905, 11.3561)
  line L830 (-38.905, 11.3561) -> (-39.1417, 11.344)
  line L831 (-38.3425, 17.1764) -> (-38.5928, 17.3007)
  line L832 (-39.1417, 11.344) -> (-39.3842, 11.3467)
  line L833 (-39.3842, 11.3467) -> (-39.6323, 11.364)
  line L834 (-39.6323, 11.364) -> (-39.886, 11.3956)
  line L835 (-39.886, 11.3956) -> (-40.1465, 11.4361)
  line L836 (-40.4129, 11.4882) -> (-40.6845, 11.5538)
  line L837 (-40.1465, 11.4361) -> (-40.4129, 11.4882)
  line L838 (-37.1025, 16.3084) -> (-37.2761, 16.4698)
  line L839 (-40.6845, 11.5538) -> (-41.0555, 11.6234)
  line L840 (-41.0555, 11.6234) -> (-41.4341, 11.6662)
  line L841 (-41.8176, 11.6908) -> (-42.2052, 11.7005)
  line L842 (-42.2052, 11.7005) -> (-42.5962, 11.6968)
  line L843 (-42.5962, 11.6968) -> (-42.9903, 11.6809)
  line L844 (-41.4341, 11.6662) -> (-41.8176, 11.6908)
  line L845 (-36.4388, 15.4218) -> (-36.5421, 15.6124)
  line L846 (-36.2795, 15.0209) -> (-36.3516, 15.2235)
  line L847 (-36.3516, 15.2235) -> (-36.4388, 15.4218)
  line L848 (-43.387, 11.6536) -> (-43.7863, 11.6156)
  line L849 (-46.223, 11.1825) -> (-46.6346, 11.0786)
  line L850 (-45.8128, 11.2778) -> (-46.223, 11.1825)
  line L851 (-45.4041, 11.3641) -> (-45.8128, 11.2778)
  line L852 (-44.9969, 11.4412) -> (-45.4041, 11.3641)
  line L853 (-44.5914, 11.509) -> (-44.9969, 11.4412)
  line L854 (-44.1878, 11.5673) -> (-44.5914, 11.509)
  line L855 (-43.7863, 11.6156) -> (-44.1878, 11.5673)
  line L856 (-46.6346, 11.0786) -> (-47.0473, 10.9659)
  line L857 (-47.0473, 10.9659) -> (-47.4611, 10.8448)
  line L858 (-47.4611, 10.8448) -> (-47.8758, 10.7152)
  line L859 (-47.8758, 10.7152) -> (-48.2914, 10.5774)
  line L860 (-48.2914, 10.5774) -> (-48.7077, 10.4313)
  line L861 (-48.7077, 10.4313) -> (-48.7824, 10.0761)
  line L862 (-48.7824, 10.0761) -> (-48.8546, 9.7203)
  line L863 (-48.8546, 9.7203) -> (-48.9241, 9.3639)
  line L864 (-48.9241, 9.3639) -> (-48.9911, 9.0071)
  line L865 (-48.9911, 9.0071) -> (-49.0554, 8.6498)
  line L866 (-42.9903, 11.6809) -> (-43.387, 11.6536)
  line L867 (-36.2262, 14.8073) -> (-36.2795, 15.0209)
  line L868 (-40.4408, 18.6855) -> (-40.7272, 18.9615)
  line L869 (-40.1491, 18.4201) -> (-40.4408, 18.6855)
  line L870 (-39.852, 18.1659) -> (-40.1491, 18.4201)
  line L871 (-39.5489, 17.9241) -> (-39.852, 18.1659)
  line L872 (-39.2392, 17.6965) -> (-39.5489, 17.9241)
  line L873 (-38.9217, 17.4859) -> (-39.2392, 17.6965)
  line L874 (-40.7272, 18.9615) -> (-41.0086, 19.2472)
  line L875 (-41.0086, 19.2472) -> (-41.2851, 19.5423)
  line L876 (-42.8453, 21.4895) -> (-43.0891, 21.841)
  line L877 (-42.5969, 21.1453) -> (-42.8453, 21.4895)
  line L878 (-42.3439, 20.8086) -> (-42.5969, 21.1453)
  line L879 (-42.0862, 20.4798) -> (-42.3439, 20.8086)
  line L880 (-41.8239, 20.1589) -> (-42.0862, 20.4798)
  line L881 (-41.5569, 19.8464) -> (-41.8239, 20.1589)
  line L882 (-41.2851, 19.5423) -> (-41.5569, 19.8464)
  line L883 (-43.0891, 21.841) -> (-43.3282, 22.1998)
  line L884 (-43.5626, 22.5656) -> (-43.7924, 22.9383)
  line L885 (-43.7924, 22.9383) -> (-44.0174, 23.3178)
  line L886 (-44.0174, 23.3178) -> (-43.8463, 23.638)
  line L887 (-43.8463, 23.638) -> (-43.6728, 23.957)
  line L888 (-43.6728, 23.957) -> (-43.4971, 24.2746)
  line L889 (-43.4971, 24.2746) -> (-43.319, 24.591)
  line L890 (-43.319, 24.591) -> (-43.1386, 24.9061)
  line L891 (-43.3282, 22.1998) -> (-43.5626, 22.5656)
  line L892 (-36.1896, 14.5898) -> (-36.2262, 14.8073)
  line L893 (-36.1751, 14.3579) -> (-36.1896, 14.5898)
  line L894 (-36.1824, 14.1175) -> (-36.1751, 14.3579)
  line L895 (-36.2227, 13.8474) -> (-36.1824, 14.1175)
  line L896 (-36.3174, 13.5133) -> (-36.2227, 13.8474)
  line L897 (-36.3367, 13.4614) -> (-36.3174, 13.5133)
  line L898 (-36.3559, 13.4094) -> (-36.3367, 13.4614)
  line L899 (-36.375, 13.3574) -> (-36.3559, 13.4094)
  line L900 (-36.3941, 13.3053) -> (-36.375, 13.3574)
  line L901 (-36.4131, 13.2533) -> (-36.3941, 13.3053)
  line L902 (-39.6781, 2.1727) -> (-39.8523, 2.3033)
  line L903 (-39.8523, 2.3033) -> (-40.0379, 2.4272)
  line L904 (-40.0379, 2.4272) -> (-40.2348, 2.5371)
  line L905 (-40.2348, 2.5371) -> (-40.4428, 2.6351)
  line L906 (-40.661, 2.7274) -> (-40.8898, 2.8078)
  line L907 (-40.8898, 2.8078) -> (-41.1289, 2.8764)
  line L908 (-41.1289, 2.8764) -> (-41.3781, 2.9334)
  line L909 (-41.3781, 2.9334) -> (-41.6367, 2.9845)
  line L910 (-41.6367, 2.9845) -> (-41.9049, 3.0266)
  line L911 (-38.75, 0) -> (-38.75, -0.0554)
  line L912 (-38.75, -0.0554) -> (-38.7498, -0.1108)
  line L913 (-38.7498, -0.1108) -> (-38.7496, -0.1663)
  line L914 (-38.7496, -0.1663) -> (-38.7494, -0.2217)
  line L915 (-42.1825, 3.0578) -> (-42.555, 3.1194)